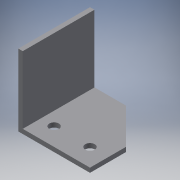
# Autodesk Inventor part: angle gusset 2
Saved by Autodesk Inventor 2016 (Build 200138000, 138)
## iProperties
Created: 2016-02-04
Part Number: angle gusset 2
Material: Generic
Document SubType Name: Modeling
Designer: gus
Density: 1 g/cm^3
Appearance: Default
Author: gus
Autodesk Inventor part; units mm, degrees
ref_plane "YZ Plane" through (0, 0, 0) normal (1, 0, 0) x (0, 1, 0)
ref_plane "XZ Plane" through (0, 0, 0) normal (0, 1, 0) x (-1, 0, 0)
ref_plane "XY Plane" through (0, 0, 0) normal (0, 0, 1) x (1, 0, 0)
sketch "Sketch1" plane through (0, 0, 0) normal (0, 0, 1) x (1, 0, 0)
  line L0 (0, 0) -> (0, 50.8)
  line L1 (0, 50.8) -> (3.175, 50.8)
  line L2 (3.175, 50.8) -> (3.175, 3.175)
  line L3 (3.175, 3.175) -> (50.8, 3.175)
  line L4 (50.8, 3.175) -> (50.8, 0)
  line L5 (50.8, 0) -> (0, 0)
  dimension "d0" = 50.8
  dimension "d1" = 3.175
  dimension "d2" = 47.625
  dimension "d3" = 47.625
  constraints: 12 end point, 4 perpendicular, 1 parallel, 1 vertical
  measures "d0" distance of L0.start L0.end
  measures "d1" distance of L0.end L1.end
  measures "d2" distance of L1.end L2.end
  measures "d3" distance of L2.end L3.end
extrude "Extrusion1" add sketch "Sketch1" along normal blind 50.8
sketch "Sketch2" plane through (3.175, 3.175, 0) normal (0, 1, 0) x (1, 0, 0)
  line L0 (47.625, 0) -> (47.625, -50.8) projected
  line L1 (47.625, -25.4) -> (22.225, 0)
  line L2 (47.625, 0) -> (-3.175, 0) projected
  line L3 (0, 0) -> (0, -50.8) projected
  line L4 (47.625, -25.4) -> (47.625, 0)
  line L5 (22.225, 0) -> (47.625, 0)
  circle A0 centre (34.925, -38.1) radius 3.3734
  circle A1 centre (9.525, -38.1) radius 3.3734
  line L6 (47.625, -50.8) -> (0, -50.8) projected
  dimension "d6" = 22.225
  dimension "d7" = 6.7469
  dimension "d8" = 6.7469
  dimension "d9" = 12.7
  dimension "d10" = 12.7
  dimension "d11" = 12.7
  dimension "d12" = 38.1
  constraints: 6 end point, 2 centre point, 2 midpoint, 1 collinear, 1 perpendicular
  measures "d6" distance from line of L3 L1.end
  measures "d7" diameter of A0
  measures "d8" diameter of A1
  measures "d9" distance from line of L0 A0.centre
  measures "d10" distance from line of L6 A0.centre
  measures "d11" distance from line of L6 A1.centre
  measures "d12" distance from line of L0 A1.centre
extrude "Extrusion2" cut sketch "Sketch2" against normal blind 50.8 contours L0 L1 L2 | A0 | A1
sketch "Sketch3" plane through (3.175, 3.175, 0) normal (1, 0, 0) x (0, 0, -1)
  circle A0 centre (-38.1, 9.525) radius 3.3734
  circle A1 centre (-12.7, 34.925) radius 3.3734
  line L0 (0, 47.625) -> (-50.8, 47.625) projected
  line L1 (0, 47.625) -> (0, 0) projected
  line L2 (-25.4, -3.175) -> (-50.8, -3.175) projected
  line L3 (-50.8, 0) -> (-50.8, 47.625) projected
  point P0 (0, -3.175)
  dimension "d15" = 6.7469
  dimension "d16" = 6.7469
  dimension "d17" = 12.7
  dimension "d18" = 12.7
  dimension "d19" = 12.7
  dimension "d20" = 12.7
  constraints: 2 centre point
  measures "d15" diameter of A0
  measures "d16" diameter of A1
  measures "d17" distance from line of L0 A1.centre
  measures "d18" distance from line of L1 A1.centre
  measures "d19" distance from line of L2 A0.centre
  measures "d20" distance from line of L3 A0.centre
extrude "Extrusion3" cut sketch "Sketch3" against normal blind 3.175
body "Solid1"
